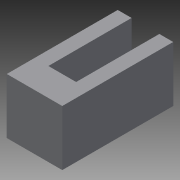
# Autodesk Inventor part: rod grabber
Saved by Autodesk Inventor 2015 (Build 190159000, 159)
## iProperties
Created: 2015-04-10
Part Number: rod grabber
Material: Generic
Document SubType Name: Modeling
Designer: WASHHSST
Density: 1 g/cm^3
Appearance: Default
Author: WASHHSST
Autodesk Inventor part; units mm, degrees
ref_plane "YZ Plane" through (0, 0, 0) normal (1, 0, 0) x (0, 1, 0)
ref_plane "XZ Plane" through (0, 0, 0) normal (0, 1, 0) x (-1, 0, 0)
ref_plane "XY Plane" through (0, 0, 0) normal (0, 0, 1) x (1, 0, 0)
sketch "Sketch1" plane through (0, 0, 0) normal (0, 1, 0) x (-1, 0, 0)
  line L0 (0, 0) -> (12.7, 0)
  line L1 (12.7, 0) -> (12.7, -25.4)
  line L2 (12.7, -25.4) -> (0, -25.4)
  line L3 (0, -25.4) -> (0, 0)
  line L4 (9.525, -25.4) -> (9.525, -6.35)
  line L5 (9.525, -6.35) -> (3.175, -6.35)
  line L6 (3.175, -6.35) -> (3.175, -25.4)
  dimension "d0" = 12.7
  dimension "d1" = 25.4
  dimension "d4" = 19.05
  dimension "d16" = 6.35
  dimension "d17" = 3.175
  dimension "d18" = 3.175
  constraints: 14 end point, 3 perpendicular, 2 parallel, 2 point on line, 1 horizontal, 1 vertical
  measures "d0" distance of L1.end L2.end
  measures "d1" distance of L0.end L1.end
  measures "d4" distance between parallel lines of L2 L5
  measures "d16" distance between parallel lines of L6 L4
  measures "d17" distance between parallel lines of L6 L3
  measures "d18" distance between parallel lines of L4 L1
extrude "Extrusion1" add sketch "Sketch1" along normal blind 12.7 contours L0 L1 L2 L4 L5 L6 L3
body "Solid1"
